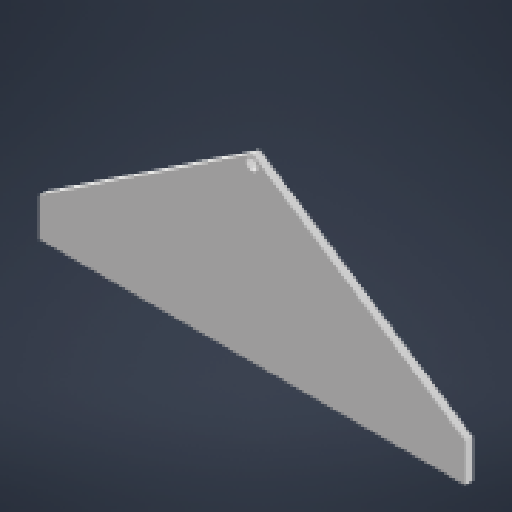
# Autodesk Inventor part: Pieza7
Saved by Autodesk Inventor 2026.1 (Build 301233020, 233B)
## iProperties
Created: 2026-05-06
Part Number: Pieza7
Material: Genérico
Document SubType Name: Modeling
Designer: OlmesTech
Density: 1 g/cm^3
Appearance: Valor por defecto
Author: OlmesTech
Autodesk Inventor part; units mm, degrees
ref_plane "YZ Plane" through (0, 0, 0) normal (1, 0, 0) x (0, 1, 0)
ref_plane "XZ Plane" through (0, 0, 0) normal (0, 1, 0) x (-1, 0, 0)
ref_plane "XY Plane" through (0, 0, 0) normal (0, 0, 1) x (1, 0, 0)
sketch "Boceto1" plane through (0, 0, 0) normal (0, 0, 1) x (1, 0, 0)
  arc A0 (-1.5, 113.1763) -> (1.5, 113.1763) centre (0, 113.1763) ccw
  line L0 (0, 113.1763) -> (0, 116.1763)
  line L1 (-75, 45) -> (75, 45) projected
  line L2 (75, 45) -> (85, 45)
  line L3 (-75, 45) -> (-85, 45)
  line L4 (0, 117.735) -> (-0.0114, 117.7429)
  line L5 (-85, 55) -> (0, 111.6763) projected
  line L6 (0, 111.6763) -> (85, 55) projected
  line L7 (-2.22, 113.8018) -> (0.2156, 115.4258) projected
  line L8 (1.8799, 112.9298) -> (0.2156, 115.4258) projected
  line L9 (-0.5557, 111.3058) -> (1.8799, 112.9298) projected
  line L10 (1.8799, 112.9298) -> (0.2156, 115.4258) projected
  line L11 (-2.22, 113.8018) -> (0.2156, 115.4258) projected
  line L12 (-0.5557, 111.3058) -> (-2.22, 113.8018) projected
  line L13 (-2.22, 113.8018) -> (1.8799, 112.9298)
  line L14 (-0.5557, 111.3058) -> (0.2156, 115.4258)
  circle A1 centre (-0.17, 113.3658) radius 2.0958
  line L15 (85, 45) -> (85, 59.843)
  line L16 (-85, 45) -> (-85, 59.843)
  circle A2 centre (-0.17, 113.3658) radius 2.1904
  line L17 (0, 117.0317) -> (-85, 60.3554) projected
  line L18 (85, 60.3554) -> (0, 117.0317) projected
  line L19 (-85, 60.3554) -> (-85, 45) projected
  line L20 (85, 45) -> (85, 60.3554) projected
  point P0 (0, 0)
  point P1 (96.4858, 46.8907)
  point P2 (-94.6783, 48.1668)
  point P3 (-94.6783, 45)
  point P4 (96.4858, 45)
  dimension "d0" = 3
  constraints: 16 end point, 3 point on line, 2 centre point, 2 coincident, 2 horizontal, 2 point on circle, 2 vertical, 1 midpoint, 1 parallel, 4 other
  measures "d0" distance of L0.start L0.end
extrude "Extrusión1" add sketch "Boceto1" along normal blind 3 contours A2 L6 L15 L2 L1 L3 L16 L5 | L5 L16 L19 L17 L18 L20 L15 L6 A2
